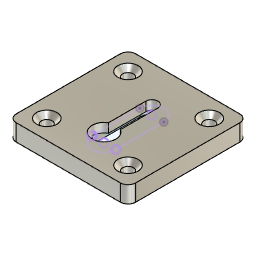
HangerPlate v12 (Autodesk Fusion 360 design; units mm, degrees)
Autodesk Fusion 360 part; units mm, degrees
note: some values were not read from the file. Set by a fixed rule: which sketch regions a step uses.
sketch "Sketch1" plane through (0, 0, 0) normal (0, 0, 1) x (1, 0, 0)
  line L0 (0, 0) -> (50, 0)
  line L1 (50, 0) -> (50, 50)
  line L2 (50, 50) -> (0, 50)
  line L3 (0, 50) -> (0, 0)
  circle A0 centre (8, 42) radius 2.25
  line L4 (8, 42) -> (42, 42) construction
  line L5 (42, 42) -> (42, 8) construction
  line L6 (42, 8) -> (8, 8) construction
  line L7 (8, 8) -> (8, 42) construction
  circle A1 centre (8, 8) radius 2.25
  circle A2 centre (42, 42) radius 2.25
  circle A3 centre (42, 8) radius 2.25
  circle A4 centre (25, 15) radius 5
  line L8 (25, 15) -> (25, 35) construction
  circle A5 centre (25, 35) radius 5
  circle A6 centre (25, 35) radius 2.5
  circle A7 centre (25, 20) radius 2.5
  line L9 (27.5, 15) -> (27.5, 35)
  line L10 (22.5, 15) -> (22.5, 35)
  line L11 (30, 15) -> (30, 35)
  line L12 (20, 15) -> (20, 35)
  dimension "d1" = 50
  dimension "d2" = 4.5
  dimension "d3" = 8
  dimension "d4" = 8
  dimension "d5" = 8
  dimension "d6" = 8
  dimension "d7" = 4.5
  dimension "d8" = 4.5
  dimension "d9" = 4.5
  dimension "d10" = 10
  dimension "d11" = 20
  dimension "d13" = 15
  dimension "d14" = 10
  dimension "d15" = 5
  dimension "d16" = 5
  dimension "d17" = 2.5
  dimension "d18" = -2.5
  dimension "d19" = 5
  dimension "d20" = -5
  constraint horizontal L0
  constraint vertical L1
  constraint horizontal L2
  constraint vertical L3
  constraint coincident L0.start L3.end
  constraint horizontal L4
  constraint vertical L5
  constraint horizontal L6
  constraint vertical L7
  constraint coincident A0.centre L4.start
  constraint coincident L6.end L7.start
  constraint coincident L4.end L5.start
  constraint coincident L5.end L6.start
  constraint coincident A4.centre L8.start
  constraint vertical L8
  constraint coincident L8.end A5.centre
  constraint concentric A5 A6
  constraint coincident L8 A7.centre
  constraint coincident A4 A7.centre
  measures "d1" distance of L0.start L2.end
  measures "d2" diameter of A0
  measures "d3" distance of L2 A0.centre
  measures "d4" distance of L3 A0.centre
  measures "d5" distance of L1 L5
  measures "d6" distance of L0 L6
  measures "d7" diameter of A1
  measures "d8" diameter of A2
  measures "d9" diameter of A3
  measures "d10" diameter of A4
  measures "d11" distance of A4.centre L8.end
  measures "d13" distance of L0 A4.centre
  measures "d14" diameter of A5
  measures "d15" diameter of A6
  measures "d16" diameter of A7
extrude "Extrude1" add sketch "Sketch1" along normal blind 7 contours L0 L1 L2 L3 | A4 A5 L10 L12 | A4 A5 L9 L11 | A5 A6 L9 L10 picked at (20.8519, 34.7516)
extrude "Extrude2" cut sketch "Sketch1" along normal blind 3.175 contours A4 A5 L10 L12 | A4 A5 L9 L11 | A5 A6 L9 L10 picked at (20.8519, 34.7516)
fillet "Fillet1" radius 3.175 4 edges at (0, 0, 3.5) (50, 0, 3.5) (50, 50, 3.5) (0, 50, 3.5)
chamfer "Chamfer1" distance 2 angle 45 4 edges at (5.9023, 42.8136, 7) (5.9023, 8.8136, 7) (39.9023, 8.8136, 7) (39.9023, 42.8136, 7)
sketch "Sketch2" plane through (0, 0, 3.175) normal (0, 0, -1) x (1, 0, 0)
  line L0 (22.5, -35) -> (22.5, -19.3301)
  arc A0 (20, -15) -> (22.5, -19.3301) centre (25, -15) ccw
  line L1 (20, -15) -> (20, -35)
  arc A1 (20, -35) -> (30, -35) centre (25, -35) ccw
  line L2 (30, -35) -> (30, -15)
  arc A2 (27.5, -19.3301) -> (30, -15) centre (25, -15) ccw
  line L3 (27.5, -19.3301) -> (27.5, -35)
  arc A3 (22.5, -35) -> (27.5, -35) centre (25, -35) ccw
  line L4 (20, -35) -> (20, -15)
  arc A4 (30, -15) -> (20, -15) centre (25, -15) ccw
  line L5 (30, -15) -> (30, -35)
  arc A5 (20, -35) -> (30, -35) centre (25, -35) ccw
